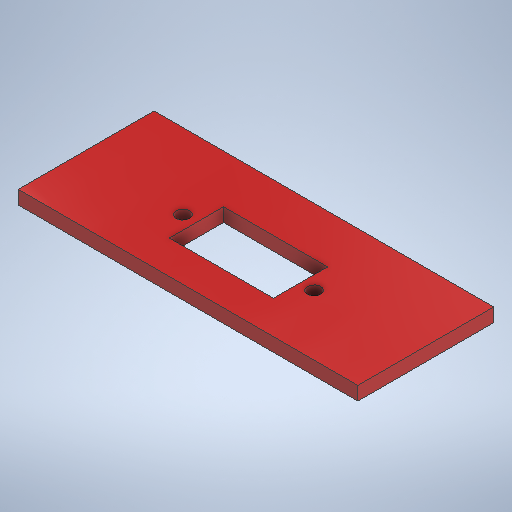
# Autodesk Inventor part: étage_devant
Saved by Autodesk Inventor 2025.1 (Build 291241000, 241)
## iProperties
Created: 2024-11-30
Part Number: étage_devant
Material: Générique
Document SubType Name: Modeling
Designer: yasmi
Density: 1 g/cm^3
Appearance: Par défaut
Author: yasmi
Autodesk Inventor part; units mm, degrees
ref_plane "YZ Plane" through (0, 0, 0) normal (1, 0, 0) x (0, 1, 0)
ref_plane "XZ Plane" through (0, 0, 0) normal (0, 1, 0) x (-1, 0, 0)
ref_plane "XY Plane" through (0, 0, 0) normal (0, 0, 1) x (1, 0, 0)
sketch "Esquisse1" plane through (0, 0, 0) normal (0, 1, 0) x (-1, 0, 0)
  line L0 (9, 14) -> (-66, 14)
  line L1 (-66, 14) -> (-66, -16)
  line L2 (-66, -16) -> (9, -16)
  line L3 (9, -16) -> (9, 14)
  line L4 (-17, 6.6599) -> (-40, 6.6599)
  line L5 (-40, 6.6599) -> (-40, -5.3401)
  line L6 (-40, -5.3401) -> (-17, -5.3401)
  line L7 (-17, -5.3401) -> (-17, 6.6599)
  circle A0 centre (-14, 0.6599) radius 1.5
  circle A1 centre (-43, 0.6599) radius 1.5
  line L8 (17, -5.3401) -> (-82, -5.3401)
  point P0 (0, 0)
  point P1 (-17, 0.6599)
  dimension "d0" = 75
  dimension "d1" = 30
  dimension "d2" = 23
  dimension "d3" = 12
  dimension "d4" = 3
  dimension "d5" = 3
  dimension "d6" = 3
  dimension "d7" = 3
  dimension "d8" = 6
  dimension "d9" = 6
  dimension "d10" = 26
  constraints: 18 end point, 4 parallel, 2 centre point, 2 horizontal, 2 perpendicular, 2 point on line, 1 midpoint
  measures "d0" distance of L2.end L1.end
  measures "d1" distance of L0.end L1.end
  measures "d2" distance of L6.end L5.end
  measures "d3" distance of L4.end L5.end
  measures "d4" diameter of A0
  measures "d5" diameter of A1
  measures "d6" distance of A0.centre point (-17, 0.66)
  measures "d7" distance from line of L5 A1.centre
  measures "d8" distance from line of L8 A0.centre
  measures "d9" distance from line of L8 A1.centre
  measures "d10" distance between parallel lines of L3 L7
extrude "Extrusion1" add sketch "Esquisse1" along normal blind 3 contours L3 L8 L7 L4 L5 L1 L0 | L3 L2 L1 L8 L6
